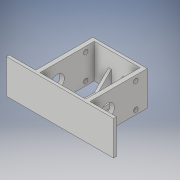
# Autodesk Inventor part: engine_mount
Saved by Autodesk Inventor 2019.4 (Build 234330000, 330)
## iProperties
Created: 2020-04-09
Part Number: engine_mount
Material: Типовые
Document SubType Name: Modeling
Designer: NoName
Density: 1 g/cm^3
Appearance: По умолчанию
Author: NoName
Autodesk Inventor part; units mm, degrees
ref_plane "YZ Plane" through (0, 0, 0) normal (1, 0, 0) x (0, 1, 0)
ref_plane "XZ Plane" through (0, 0, 0) normal (0, 1, 0) x (-1, 0, 0)
ref_plane "XY Plane" through (0, 0, 0) normal (0, 0, 1) x (1, 0, 0)
sketch "Эскиз1" plane through (0, 0, 0) normal (0, 1, 0) x (-1, 0, 0)
  line L0 (19, -20) -> (-19, -20)
  line L1 (-19, -20) -> (-19, 20)
  line L2 (-19, 20) -> (19, 20) construction
  line L3 (19, 20) -> (19, -20)
  line L4 (37.5, 20) -> (-37.5, 20) construction
  line L5 (-37.5, 20) -> (-37.5, 22)
  line L6 (-37.5, 22) -> (37.5, 22)
  line L7 (37.5, 22) -> (37.5, 20)
  line L8 (19, 20) -> (37.5, 20)
  line L9 (-19, 20) -> (-37.5, 20)
  line L10 (16, -18) -> (-16, -18)
  line L11 (-16, -18) -> (-16, 20)
  line L12 (-16, 20) -> (16, 20)
  line L13 (16, 20) -> (16, -18)
  point P0 (0, 0)
  point P1 (-19, 0)
  point P2 (0, -20)
  point P3 (0, 20)
  point P4 (0, -18)
  dimension "d0" = 38
  dimension "d1" = 40
  dimension "d2" = 75
  dimension "d3" = 2
  dimension "d13" = 3
  dimension "d14" = 2
  constraints: 28 end point, 6 parallel, 5 midpoint, 3 horizontal, 3 perpendicular, 2 collinear, 2 vertical alignment, 1 horizontal alignment, 1 point on line
  measures "d0" distance between parallel lines of L1 L3
  measures "d1" distance between parallel lines of L2 L0
  measures "d2" distance between parallel lines of L5 L7
  measures "d3" distance between parallel lines of L4 L6
  measures "d13" distance between parallel lines of L3 L13
  measures "d14" distance between parallel lines of L0 L10
extrude "Выдавливание1" add sketch "Эскиз1" along normal blind 24
sketch "Эскиз2" plane through (19, 0, 20) normal (1, 0, 0) x (0, 0, -1)
  line L0 (0, 0) -> (0, 24) projected
  line L1 (40, 0) -> (40, 24) projected
  line L2 (40, 0) -> (0, 0) projected
  point P0 (20, 0)
  point P1 (32, 20.5)
  point P2 (32, 3)
  dimension "d15" = 17.5
  dimension "d16" = 32
  dimension "d17" = 3
  constraints: 1 vertical alignment
  measures "d15" distance of point (32, 3) point (32, 20.5)
  measures "d16" distance from line of L0 point (32, 20.5)
  measures "d17" distance from line of L2 point (32, 3)
hole "Отверстие1" at (19, 20.5, -12) at (19, 3, -12) direction (-1, 0, 0) diameter 3.2 end through all
sketch "Эскиз3" plane through (19, 0, 20) normal (1, 0, 0) x (0, 0, -1)
  circle A0 centre (12, 12) radius 12 construction
  line L0 (0, 24) -> (40, 24) projected
  line L1 (40, 0) -> (0, 0) projected
  line L2 (0, 0) -> (0, 24) projected
  circle A1 centre (12, 12) radius 5
  point P0 (20, 0)
  dimension "d18" = 10
  constraints: 3 tangent, 2 centre point, 1 coincident
  measures "d18" diameter of A1
extrude "Выдавливание2" cut sketch "Эскиз3" against normal through all
sketch "Эскиз4" plane through (0, 0, 0) normal (0, -1, 0) x (1, 0, 0)
  line L0 (16, -18) -> (-16, -18) projected
  line L1 (-16, 20) -> (16, 20) projected
  line L2 (6, -18) -> (-6, -18)
  line L3 (-6, -18) -> (-6, 20)
  line L4 (-6, 20) -> (6, 20)
  line L5 (6, 20) -> (6, -18)
  point P0 (0, 0)
  point P1 (0, -18)
  point P2 (0, 20)
  point P3 (0, -18)
  point P4 (0, 20)
  point P5 (0, -18)
  dimension "d26" = 12
  constraints: 8 end point, 6 midpoint, 2 parallel, 2 point on line, 1 horizontal, 1 perpendicular
  measures "d26" distance between parallel lines of L3 L5
extrude "Выдавливание3" add sketch "Эскиз4" against normal blind 3
sketch "Эскиз5" plane through (6, 0, 20) normal (1, 0, 0) x (0, 0, -1)
  line L0 (0, 0) -> (0, 24) projected
  line L1 (0, 13) -> (10, 3)
  line L2 (38, 3) -> (0, 3) projected
  line L3 (40, 24) -> (0, 24) projected
  line L4 (19, 24) -> (19, 3)
  line L5 (38, 13) -> (28, 3)
  line L6 (38, 13) -> (38, 3)
  line L7 (28, 3) -> (38, 3)
  line L8 (10, 3) -> (0, 3)
  line L9 (0, 3) -> (0, 13)
  point P0 (20, 0)
  dimension "d27" = 45
  dimension "d28" = 10
  constraints: 14 end point, 3 point on line, 2 collinear, 2 perpendicular, 2 symmetric about line, 1 midpoint, 1 vertical
  measures "d27" angle of L0 L1
  measures "d28" distance of L2.end L1.end
extrude "Выдавливание4" add sketch "Эскиз5" against normal blind 2 contours L5 L6 L2 | L0 L1 L2
mirror "Зеркальное отражение1" about plane through (0, 0, 0) normal (1, 0, 0) of "Выдавливание4"
sketch "Эскиз6" plane through (0, 3, 0) normal (0, 1, 0) x (1, 0, 0)
  line L0 (-6, 8) -> (-6, -10) projected
  line L1 (6, -20) -> (6, 18) projected
  line L2 (-16, 18) -> (-16, -20) projected
  line L3 (-16, -1) -> (16, -1)
  line L4 (16, 18) -> (16, -20) projected
  point P0 (0, 0)
  point P1 (0, -16)
  point P2 (0, 14)
  dimension "d38" = 30
  constraints: 2 end point, 2 midpoint, 2 vertical alignment, 1 symmetric about line
  measures "d38" distance of point (0, 14) point (0, -16)
hole "Отверстие2" at (0, 3, 16) at (0, 3, -14) direction (0, -1, 0) diameter 3.2 end through all
